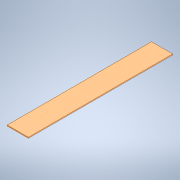
# Autodesk Inventor part: Bovenkant
Saved by Autodesk Inventor 2021 (Build 250183000, 183)
## iProperties
Created: 2021-03-18
Part Number: Bovenkant
Material: Wood (Cherry)
Document SubType Name: Modeling
Designer: ZiweZhang
Density: 0.63 g/cm^3
Appearance: Cherry - Natural Low Gloss
Author: ZiweZhang
Autodesk Inventor part; units mm, degrees
ref_plane "YZ Plane" through (0, 0, 0) normal (1, 0, 0) x (0, 1, 0)
ref_plane "XZ Plane" through (0, 0, 0) normal (0, 1, 0) x (-1, 0, 0)
ref_plane "XY Plane" through (0, 0, 0) normal (0, 0, 1) x (1, 0, 0)
sketch "Sketch1" plane through (0, 0, 0) normal (0, 1, 0) x (-1, 0, 0)
  line L0 (-71, 485) -> (71, 485)
  line L1 (71, 485) -> (71, -485)
  line L2 (71, -485) -> (-71, -485)
  line L3 (-71, -485) -> (-71, 485)
  line L4 (-71, 485) -> (71, -485) construction
  line L5 (71, 485) -> (-71, -485) construction
  point P0 (0, 0)
  dimension "d0" = 142
  dimension "d1" = 970
  constraints: 12 end point, 2 midpoint, 2 parallel, 1 horizontal, 1 perpendicular
  measures "d0" distance of L1.end L2.end
  measures "d1" distance of L0.end L1.end
extrude "Extrusion1" add sketch "Sketch1" along normal blind 6
body "Solid1"
